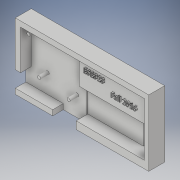
# Autodesk Inventor part: case2
Saved by Autodesk Inventor 2017 (Build 210142000, 142)
## iProperties
Created: 2016-12-01
Part Number: case2
Material: Generic
Document SubType Name: Modeling
Designer: SDL
Density: 1 g/cm^3
Appearance: Default
Author: SDL
Autodesk Inventor part; units mm, degrees
ref_plane "YZ Plane" through (0, 0, 0) normal (1, 0, 0) x (0, 1, 0)
ref_plane "XZ Plane" through (0, 0, 0) normal (0, 1, 0) x (-1, 0, 0)
ref_plane "XY Plane" through (0, 0, 0) normal (0, 0, 1) x (1, 0, 0)
sketch "Sketch3" plane through (0, 0, 0) normal (0, 0, 1) x (1, 0, 0)
  line L0 (0, 0) -> (125, 0)
  line L1 (125, 0) -> (125, 62)
  line L2 (125, 62) -> (0, 62)
  line L3 (0, 62) -> (0, 0)
  dimension "d0" = 125
  dimension "d1" = 62
  constraints: 8 end point, 2 parallel, 1 horizontal, 1 perpendicular
  measures "d0" distance of L2.end L1.end
  measures "d1" distance of L1.end L0.end
extrude "Extrusion1" add sketch "Sketch3" along normal blind 15
sketch "Sketch4" plane through (0, 0, 15) normal (0, 0, 1) x (1, 0, 0)
  line L0 (0, 62) -> (0, 0) projected
  line L1 (125, 0) -> (125, 62) projected
  line L2 (5, 57) -> (57, 57)
  line L3 (57, 57) -> (57, 5)
  line L4 (57, 5) -> (5, 5)
  line L5 (5, 5) -> (5, 57)
  line L6 (4, 57) -> (56, 5) construction
  line L7 (56, 57) -> (4, 5) construction
  dimension "d4" = 52
  dimension "d5" = 52
  constraints: 12 end point, 2 parallel, 1 horizontal, 1 perpendicular
  measures "d4" distance of L3.end L4.end
  measures "d5" distance of L2.end L3.end
extrude "Extrusion2" cut sketch "Sketch4" against normal blind 10
sketch "Sketch5" plane through (0, 0, 15) normal (0, 0, 1) x (1, 0, 0)
  line L0 (57, 57) -> (57, 5) projected
  line L1 (57, 5) -> (57, 7)
  line L2 (0, 0) -> (125, 0) projected
  line L3 (57, 7) -> (121, 7)
  line L4 (121, 7) -> (121, 33.5)
  line L5 (121, 33.5) -> (57, 33.5)
  line L6 (57, 33.5) -> (57, 7)
  dimension "d9" = 2
  dimension "d10" = 64
  dimension "d11" = 26.5
  constraints: 10 end point, 2 parallel, 2 perpendicular, 1 horizontal
  measures "d9" distance of L0.end L1.end
  measures "d10" distance of L5.end L4.end
  measures "d11" distance of L4.end L3.end
extrude "Extrusion3" cut sketch "Sketch5" against normal blind 10
sketch "Sketch6" plane through (0, 0, 15) normal (0, 0, 1) x (1, 0, 0)
  line L0 (121, 7) -> (57, 7) projected
  line L1 (57, 33.5) -> (121, 33.5) projected
  line L2 (121, 7) -> (109, 7)
  line L3 (109, 7) -> (109, 33.5)
  line L4 (109, 33.5) -> (121, 33.5)
  line L5 (121, 33.5) -> (121, 7)
  point P0 (0, 0)
  dimension "d14" = 12
  constraints: 8 end point, 2 parallel, 1 horizontal, 1 perpendicular, 1 point on line
  measures "d14" distance of L3.end L4.end
extrude "Extrusion4" cut sketch "Sketch6" against normal blind 15
sketch "Sketch7" plane through (0, 0, 15) normal (0, 0, 1) x (1, 0, 0)
  line L0 (109, 7) -> (57, 7) projected
  line L1 (109, 33.5) -> (109, 7) projected
  line L2 (57, 7) -> (109, 7)
  line L3 (109, 7) -> (109, 33.5)
  line L4 (109, 33.5) -> (57, 33.5)
  line L5 (57, 33.5) -> (57, 7)
  point P0 (0, 0)
  constraints: 8 end point, 2 parallel, 1 horizontal, 1 perpendicular
extrude "Extrusion5" cut sketch "Sketch7" against normal blind 11
sketch "Sketch8" plane through (0, 0, 5) normal (0, 0, 1) x (1, 0, 0)
  line L0 (5, 57) -> (57, 57) projected
  line L1 (57, 5) -> (5, 5) projected
  line L2 (5, 5) -> (5, 57) projected
  line L3 (57, 7) -> (57, 33.5) projected
  line L4 (6, 56) -> (56, 6) construction
  line L5 (56, 56) -> (6, 6) construction
  line L6 (6, 6) -> (20.3, 6) construction
  circle A0 centre (10.4, 53) radius 1.5
  circle A1 centre (20.3, 22.7) radius 1.5
  circle A2 centre (47.9, 18.5) radius 1.5
  point P0 (0, 0)
  point P1 (31, 31)
  dimension "d19" = 50
  dimension "d20" = 50
  dimension "d28" = 3
  dimension "d29" = 3
  dimension "d30" = 3
  constraints: 6 end point, 3 centre point, 2 midpoint, 1 horizontal
  measures "d19" distance of L4.end L5.end
  measures "d20" distance of L5.start L4.end
  measures "d28" diameter of A0
  measures "d29" diameter of A1
  measures "d30" diameter of A2
extrude "Extrusion6" add sketch "Sketch8" along normal blind 8
sketch "Sketch9" plane through (0, 0, 15) normal (0, 0, 1) x (1, 0, 0)
  line L0 (57, 5) -> (5, 5) projected
  line L1 (5, 5) -> (35, 5)
  line L2 (0, 0) -> (125, 0) projected
  line L3 (35, 5) -> (57, 5)
  line L4 (57, 5) -> (57, 0)
  line L5 (57, 0) -> (35, 0)
  line L6 (35, 0) -> (35, 5)
  constraints: 10 end point, 2 parallel, 2 point on line, 1 horizontal, 1 perpendicular
extrude "Extrusion7" cut sketch "Sketch9" against normal blind 10
sketch "Sketch10" plane through (0, 0, 15) normal (0, 0, 1) x (1, 0, 0)
  line L0 (5, 5) -> (5, 57) projected
  line L1 (5, 57) -> (5, 20)
  line L2 (5, 20) -> (0, 20)
  line L3 (0, 62) -> (0, 0) projected
  line L4 (5, 20) -> (0, 20)
  line L5 (0, 20) -> (0, 5)
  line L6 (0, 5) -> (5, 5)
  line L7 (5, 5) -> (5, 20)
  dimension "d36" = 37
  constraints: 12 end point, 3 point on line, 2 parallel, 2 perpendicular, 1 horizontal
  measures "d36" distance of L0.end L1.end
extrude "Extrusion8" cut sketch "Sketch10" against normal blind 10
sketch "Sketch13" plane through (0, 0, 15) normal (0, 0, 1) x (1, 0, 0)
  line L0 (57, 57) -> (57, 33.5) projected
  line L1 (57, 57) -> (121, 57)
  line L2 (121, 7) -> (121, 33.5) projected
  line L3 (57, 33.5) -> (109, 33.5) projected
  line L4 (121, 57) -> (57, 57)
  line L5 (57, 57) -> (57, 33.5)
  line L6 (57, 33.5) -> (121, 33.5)
  line L7 (121, 33.5) -> (121, 57)
  point P0 (0, 0)
  constraints: 10 end point, 2 parallel, 2 perpendicular, 1 horizontal
extrude "Extrusion9" cut sketch "Sketch13" against normal blind 3
sketch "Sketch14" plane through (0, 0, 12) normal (0, 0, 1) x (1, 0, 0)
  line L0 (61.9045, 52.1131) -> (81.5918, 52.1131) construction
  line L1 (81.5918, 52.1131) -> (81.5918, 47.138) construction
  line L2 (81.5918, 47.138) -> (61.9045, 47.138) construction
  line L3 (61.9045, 47.138) -> (61.9045, 52.1131) construction
  line L4 (87.5293, 45.1674) -> (113.4964, 45.1674) construction
  line L5 (113.4964, 45.1674) -> (113.4964, 38.1257) construction
  line L6 (113.4964, 38.1257) -> (87.5293, 38.1257) construction
  line L7 (87.5293, 38.1257) -> (87.5293, 45.1674) construction
  spline S0 degree 2 poles (64.7873, 48.0985) (64.7873, 48.0393) (64.7754, 47.9525) (64.7439, 47.8973) (64.7005, 47.8697) (64.6729, 47.8697) knots 0 0 0 1 2 3 4 4 4
  line L8 (64.6729, 47.8697) -> (62.6656, 47.8697)
  spline S1 degree 2 poles (62.6656, 47.8697) (62.5946, 47.8697) (62.4605, 47.9683) (62.4605, 48.0945) knots 0 0 0 1 2 2 2
  line L9 (62.4605, 48.0945) -> (62.4605, 51.8252)
  spline S2 degree 2 poles (62.4605, 51.8252) (62.4605, 51.9514) (62.5946, 52.05) (62.6656, 52.05) knots 0 0 0 1 2 2 2
  line L10 (62.6656, 52.05) -> (64.6492, 52.05)
  spline S3 degree 2 poles (64.6492, 52.05) (64.6769, 52.05) (64.7163, 52.0224) (64.7439, 51.9672) (64.7597, 51.8804) (64.7597, 51.8134) knots 0 0 0 1 2 3 4 4 4
  spline S4 degree 2 poles (64.7597, 51.8134) (64.7597, 51.7582) (64.7439, 51.6675) (64.7163, 51.6162) (64.6769, 51.5886) (64.6492, 51.5886) knots 0 0 0 1 2 3 4 4 4
  line L11 (64.6492, 51.5886) -> (63.0166, 51.5886)
  line L12 (63.0166, 51.5886) -> (63.0166, 50.2754)
  line L13 (63.0166, 50.2754) -> (64.4166, 50.2754)
  spline S5 degree 2 poles (64.4166, 50.2754) (64.4442, 50.2754) (64.4836, 50.2478) (64.5152, 50.1965) (64.527, 50.1058) (64.527, 50.0427) knots 0 0 0 1 2 3 4 4 4
  spline S6 degree 2 poles (64.527, 50.0427) (64.527, 49.9835) (64.5152, 49.9007) (64.4836, 49.8494) (64.4442, 49.8258) (64.4166, 49.8258) knots 0 0 0 1 2 3 4 4 4
  line L14 (64.4166, 49.8258) -> (63.0166, 49.8258)
  line L15 (63.0166, 49.8258) -> (63.0166, 48.3311)
  line L16 (63.0166, 48.3311) -> (64.6729, 48.3311)
  spline S7 degree 2 poles (64.6729, 48.3311) (64.7005, 48.3311) (64.7439, 48.3035) (64.7754, 48.2523) (64.7873, 48.1616) (64.7873, 48.0985) knots 0 0 0 1 2 3 4 4 4
  spline S8 degree 2 poles (67.9343, 49.041) (67.9343, 48.7492) (67.7174, 48.2878) (67.3349, 47.9683) (66.8143, 47.8066) (66.5146, 47.8066) knots 0 0 0 1 2 3 4 4 4
  spline S9 degree 2 poles (66.5146, 47.8066) (66.3016, 47.8066) (65.9428, 47.8776) (65.6628, 47.9801) (65.4735, 48.0906) (65.3985, 48.1655) (65.3631, 48.2838) (65.3631, 48.3863) knots 0 0 0 1 2 3 4 5 6 6 6
  spline S10 degree 2 poles (65.3631, 48.3863) (65.3631, 48.4573) (65.3749, 48.552) (65.4025, 48.6072) (65.4419, 48.6309) (65.4656, 48.6309) knots 0 0 0 1 2 3 4 4 4
  spline S11 degree 2 poles (65.4656, 48.6309) (65.5129, 48.6309) (65.6785, 48.5204) (65.9349, 48.3942) (66.3016, 48.2799) (66.5383, 48.2799) knots 0 0 0 1 2 3 4 4 4
  spline S12 degree 2 poles (66.5383, 48.2799) (66.7197, 48.2799) (67.0233, 48.3785) (67.2363, 48.5559) (67.3546, 48.8162) (67.3546, 48.9818) knots 0 0 0 1 2 3 4 4 4
  spline S13 degree 2 poles (67.3546, 48.9818) (67.3546, 49.1593) (67.1929, 49.4117) (66.9287, 49.601) (66.5895, 49.7587) (66.2307, 49.9244) (65.8954, 50.1255) (65.6312, 50.3976) (65.4656, 50.7604) (65.4656, 51.0168) knots 0 0 0 1 2 3 4 5 6 7 8 8 8
  spline S14 degree 2 poles (65.4656, 51.0168) (65.4656, 51.277) (65.6549, 51.6911) (65.994, 51.9672) (66.4633, 52.1131) (66.7354, 52.1131) knots 0 0 0 1 2 3 4 4 4
  spline S15 degree 2 poles (66.7354, 52.1131) (66.8735, 52.1131) (67.1535, 52.0658) (67.4019, 51.9869) (67.5991, 51.8844) (67.6583, 51.8252) (67.678, 51.7897) (67.6898, 51.7345) (67.6977, 51.6556) (67.6977, 51.5965) knots 0 0 0 1 2 3 4 5 6 7 8 8 8
  spline S16 degree 2 poles (67.6977, 51.5965) (67.6977, 51.5373) (67.6898, 51.4466) (67.6701, 51.3835) (67.6346, 51.3559) (67.6109, 51.3559) knots 0 0 0 1 2 3 4 4 4
  spline S17 degree 2 poles (67.6109, 51.3559) (67.5754, 51.3559) (67.4216, 51.4466) (67.2047, 51.557) (66.9011, 51.6517) (66.7157, 51.6517) knots 0 0 0 1 2 3 4 4 4
  spline S18 degree 2 poles (66.7157, 51.6517) (66.5422, 51.6517) (66.2819, 51.557) (66.1123, 51.4032) (66.0295, 51.1903) (66.0295, 51.068) knots 0 0 0 1 2 3 4 4 4
  spline S19 degree 2 poles (66.0295, 51.068) (66.0295, 50.8945) (66.1912, 50.6421) (66.4594, 50.4489) (66.8025, 50.2872) (67.1574, 50.1216) (67.5005, 49.9244) (67.7687, 49.6562) (67.9343, 49.2894) (67.9343, 49.041) knots 0 0 0 1 2 3 4 5 6 7 8 8 8
  spline S20 degree 2 poles (71.0577, 48.0985) (71.0577, 48.0393) (71.0459, 47.9525) (71.0143, 47.8973) (70.9709, 47.8697) (70.9433, 47.8697) knots 0 0 0 1 2 3 4 4 4
  line L17 (70.9433, 47.8697) -> (68.936, 47.8697)
  spline S21 degree 2 poles (68.936, 47.8697) (68.865, 47.8697) (68.7309, 47.9683) (68.7309, 48.0945) knots 0 0 0 1 2 2 2
  line L18 (68.7309, 48.0945) -> (68.7309, 51.8252)
  spline S22 degree 2 poles (68.7309, 51.8252) (68.7309, 51.9514) (68.865, 52.05) (68.936, 52.05) knots 0 0 0 1 2 2 2
  line L19 (68.936, 52.05) -> (70.9197, 52.05)
  spline S23 degree 2 poles (70.9197, 52.05) (70.9473, 52.05) (70.9867, 52.0224) (71.0143, 51.9672) (71.0301, 51.8804) (71.0301, 51.8134) knots 0 0 0 1 2 3 4 4 4
  spline S24 degree 2 poles (71.0301, 51.8134) (71.0301, 51.7582) (71.0143, 51.6675) (70.9867, 51.6162) (70.9473, 51.5886) (70.9197, 51.5886) knots 0 0 0 1 2 3 4 4 4
  line L20 (70.9197, 51.5886) -> (69.287, 51.5886)
  line L21 (69.287, 51.5886) -> (69.287, 50.2754)
  line L22 (69.287, 50.2754) -> (70.687, 50.2754)
  spline S25 degree 2 poles (70.687, 50.2754) (70.7146, 50.2754) (70.754, 50.2478) (70.7856, 50.1965) (70.7974, 50.1058) (70.7974, 50.0427) knots 0 0 0 1 2 3 4 4 4
  spline S26 degree 2 poles (70.7974, 50.0427) (70.7974, 49.9835) (70.7856, 49.9007) (70.754, 49.8494) (70.7146, 49.8258) (70.687, 49.8258) knots 0 0 0 1 2 3 4 4 4
  line L23 (70.687, 49.8258) -> (69.287, 49.8258)
  line L24 (69.287, 49.8258) -> (69.287, 48.3311)
  line L25 (69.287, 48.3311) -> (70.9433, 48.3311)
  spline S27 degree 2 poles (70.9433, 48.3311) (70.9709, 48.3311) (71.0143, 48.3035) (71.0459, 48.2523) (71.0577, 48.1616) (71.0577, 48.0985) knots 0 0 0 1 2 3 4 4 4
  spline S28 degree 2 poles (74.3546, 49.0647) (74.3546, 48.7768) (74.1535, 48.3154) (73.7788, 47.9841) (73.2307, 47.8066) (72.8836, 47.8066) knots 0 0 0 1 2 3 4 4 4
  spline S29 degree 2 poles (72.8836, 47.8066) (72.6746, 47.8066) (72.3118, 47.8737) (72.0278, 47.9683) (71.8385, 48.0669) (71.7912, 48.1142) (71.7636, 48.1576) (71.7439, 48.2247) (71.736, 48.3154) (71.736, 48.3863) knots 0 0 0 1 2 3 4 5 6 7 8 8 8
  spline S30 degree 2 poles (71.736, 48.3863) (71.736, 48.5007) (71.7833, 48.5914) (71.8267, 48.5914) knots 0 0 0 1 2 2 2
  spline S31 degree 2 poles (71.8267, 48.5914) (71.8543, 48.5914) (72.0318, 48.4889) (72.3039, 48.3666) (72.6746, 48.2641) (72.8994, 48.2641) knots 0 0 0 1 2 3 4 4 4
  spline S32 degree 2 poles (72.8994, 48.2641) (73.1163, 48.2641) (73.4476, 48.3745) (73.6723, 48.5756) (73.7867, 48.8478) (73.7867, 49.0094) knots 0 0 0 1 2 3 4 4 4
  spline S33 degree 2 poles (73.7867, 49.0094) (73.7867, 49.1909) (73.6447, 49.4748) (73.3647, 49.6799) (72.9625, 49.7903) (72.7061, 49.7903) knots 0 0 0 1 2 3 4 4 4
  line L26 (72.7061, 49.7903) -> (72.296, 49.7903)
  spline S34 degree 2 poles (72.296, 49.7903) (72.2684, 49.7903) (72.2171, 49.814) (72.1816, 49.8652) (72.158, 49.948) (72.158, 50.0151) knots 0 0 0 1 2 3 4 4 4
  spline S35 degree 2 poles (72.158, 50.0151) (72.158, 50.0782) (72.1777, 50.157) (72.2132, 50.2044) (72.2566, 50.228) (72.2881, 50.228) knots 0 0 0 1 2 3 4 4 4
  line L27 (72.2881, 50.228) -> (72.6509, 50.228)
  spline S36 degree 2 poles (72.6509, 50.228) (72.8639, 50.228) (73.2031, 50.3385) (73.4397, 50.5475) (73.5659, 50.8354) (73.5659, 51.0128) knots 0 0 0 1 2 3 4 4 4
  spline S37 degree 2 poles (73.5659, 51.0128) (73.5659, 51.143) (73.4831, 51.3796) (73.3135, 51.557) (73.0532, 51.6556) (72.8797, 51.6556) knots 0 0 0 1 2 3 4 4 4
  spline S38 degree 2 poles (72.8797, 51.6556) (72.6943, 51.6556) (72.3788, 51.5413) (72.1343, 51.4151) (71.9726, 51.3007) (71.9411, 51.3007) knots 0 0 0 1 2 3 4 4 4
  spline S39 degree 2 poles (71.9411, 51.3007) (71.9174, 51.3007) (71.8819, 51.3165) (71.8583, 51.3638) (71.8504, 51.4506) (71.8504, 51.5216) knots 0 0 0 1 2 3 4 4 4
  spline S40 degree 2 poles (71.8504, 51.5216) (71.8504, 51.5728) (71.8583, 51.6438) (71.878, 51.699) (71.9016, 51.7463) (71.9647, 51.8055) (72.1501, 51.9238) (72.4261, 52.0342) (72.785, 52.1131) (72.9901, 52.1131) knots 0 0 0 1 2 3 4 5 6 7 8 8 8
  spline S41 degree 2 poles (72.9901, 52.1131) (73.2819, 52.1131) (73.7236, 51.9632) (74.0154, 51.6911) (74.1614, 51.3125) (74.1614, 51.0838) knots 0 0 0 1 2 3 4 4 4
  spline S42 degree 2 poles (74.1614, 51.0838) (74.1614, 50.8866) (74.0588, 50.5475) (73.8577, 50.2832) (73.5659, 50.0979) (73.3766, 50.0624) knots 0 0 0 1 2 3 4 4 4
  line L28 (73.3766, 50.0624) -> (73.3766, 50.0585)
  spline S43 degree 2 poles (73.3766, 50.0585) (73.5935, 50.0348) (73.9523, 49.8652) (74.2087, 49.6049) (74.3546, 49.2579) (74.3546, 49.0647) knots 0 0 0 1 2 3 4 4 4
  spline S44 degree 2 poles (77.7422, 48.1103) (77.7422, 48.0511) (77.7264, 47.9604) (77.6988, 47.8973) (77.6476, 47.8697) (77.62, 47.8697) knots 0 0 0 1 2 3 4 4 4
  line L29 (77.62, 47.8697) -> (75.309, 47.8697)
  spline S45 degree 2 poles (75.309, 47.8697) (75.2616, 47.8697) (75.1946, 47.8934) (75.1473, 47.9447) (75.1236, 48.0432) (75.1236, 48.1142) knots 0 0 0 1 2 3 4 4 4
  spline S46 degree 2 poles (75.1236, 48.1142) (75.1236, 48.1773) (75.1354, 48.2759) (75.167, 48.3509) (75.2183, 48.4218) (75.2577, 48.4652) knots 0 0 0 1 2 3 4 4 4
  line L30 (75.2577, 48.4652) -> (76.0938, 49.3249)
  spline S47 degree 2 poles (76.0938, 49.3249) (76.3856, 49.6207) (76.7366, 50.094) (76.9259, 50.4804) (76.985, 50.7959) (76.985, 50.9379) knots 0 0 0 1 2 3 4 4 4
  spline S48 degree 2 poles (76.985, 50.9379) (76.985, 51.0759) (76.8904, 51.3244) (76.7129, 51.5097) (76.4487, 51.6201) (76.2752, 51.6201) knots 0 0 0 1 2 3 4 4 4
  spline S49 degree 2 poles (76.2752, 51.6201) (76.0701, 51.6201) (75.7467, 51.5097) (75.5022, 51.3835) (75.3405, 51.2731) (75.3011, 51.2731) knots 0 0 0 1 2 3 4 4 4
  spline S50 degree 2 poles (75.3011, 51.2731) (75.2774, 51.2731) (75.238, 51.3007) (75.2143, 51.3559) (75.2025, 51.4545) (75.2025, 51.5216) knots 0 0 0 1 2 3 4 4 4
  spline S51 degree 2 poles (75.2025, 51.5216) (75.2025, 51.5689) (75.2104, 51.6399) (75.2261, 51.6951) (75.2498, 51.7385) (75.3287, 51.8055) (75.518, 51.9238) (75.8059, 52.0342) (76.1529, 52.1131) (76.3422, 52.1131) knots 0 0 0 1 2 3 4 5 6 7 8 8 8
  spline S52 degree 2 poles (76.3422, 52.1131) (76.6459, 52.1131) (77.1033, 51.9435) (77.4031, 51.6438) (77.5529, 51.2494) (77.5529, 51.0286) knots 0 0 0 1 2 3 4 4 4
  spline S53 degree 2 poles (77.5529, 51.0286) (77.5529, 50.8275) (77.4819, 50.4292) (77.2532, 49.9678) (76.8194, 49.4038) (76.4566, 49.0331) knots 0 0 0 1 2 3 4 4 4
  line L31 (76.4566, 49.0331) -> (75.794, 48.343)
  line L32 (75.794, 48.343) -> (77.616, 48.343)
  spline S54 degree 2 poles (77.616, 48.343) (77.6436, 48.343) (77.6909, 48.3154) (77.7264, 48.2562) (77.7422, 48.1694) (77.7422, 48.1103) knots 0 0 0 1 2 3 4 4 4
  spline S55 degree 2 poles (81.0588, 49.0647) (81.0588, 48.7768) (80.8577, 48.3154) (80.4831, 47.9841) (79.9349, 47.8066) (79.5878, 47.8066) knots 0 0 0 1 2 3 4 4 4
  spline S56 degree 2 poles (79.5878, 47.8066) (79.3788, 47.8066) (79.016, 47.8737) (78.7321, 47.9683) (78.5428, 48.0669) (78.4954, 48.1142) (78.4678, 48.1576) (78.4481, 48.2247) (78.4402, 48.3154) (78.4402, 48.3863) knots 0 0 0 1 2 3 4 5 6 7 8 8 8
  spline S57 degree 2 poles (78.4402, 48.3863) (78.4402, 48.5007) (78.4876, 48.5914) (78.5309, 48.5914) knots 0 0 0 1 2 2 2
  spline S58 degree 2 poles (78.5309, 48.5914) (78.5585, 48.5914) (78.736, 48.4889) (79.0081, 48.3666) (79.3788, 48.2641) (79.6036, 48.2641) knots 0 0 0 1 2 3 4 4 4
  spline S59 degree 2 poles (79.6036, 48.2641) (79.8205, 48.2641) (80.1518, 48.3745) (80.3766, 48.5756) (80.4909, 48.8478) (80.4909, 49.0094) knots 0 0 0 1 2 3 4 4 4
  spline S60 degree 2 poles (80.4909, 49.0094) (80.4909, 49.1909) (80.349, 49.4748) (80.069, 49.6799) (79.6667, 49.7903) (79.4104, 49.7903) knots 0 0 0 1 2 3 4 4 4
  line L33 (79.4104, 49.7903) -> (79.0002, 49.7903)
  spline S61 degree 2 poles (79.0002, 49.7903) (78.9726, 49.7903) (78.9214, 49.814) (78.8859, 49.8652) (78.8622, 49.948) (78.8622, 50.0151) knots 0 0 0 1 2 3 4 4 4
  spline S62 degree 2 poles (78.8622, 50.0151) (78.8622, 50.0782) (78.8819, 50.157) (78.9174, 50.2044) (78.9608, 50.228) (78.9923, 50.228) knots 0 0 0 1 2 3 4 4 4
  line L34 (78.9923, 50.228) -> (79.3552, 50.228)
  spline S63 degree 2 poles (79.3552, 50.228) (79.5681, 50.228) (79.9073, 50.3385) (80.1439, 50.5475) (80.2701, 50.8354) (80.2701, 51.0128) knots 0 0 0 1 2 3 4 4 4
  spline S64 degree 2 poles (80.2701, 51.0128) (80.2701, 51.143) (80.1873, 51.3796) (80.0177, 51.557) (79.7574, 51.6556) (79.5839, 51.6556) knots 0 0 0 1 2 3 4 4 4
  spline S65 degree 2 poles (79.5839, 51.6556) (79.3985, 51.6556) (79.0831, 51.5413) (78.8385, 51.4151) (78.6769, 51.3007) (78.6453, 51.3007) knots 0 0 0 1 2 3 4 4 4
  spline S66 degree 2 poles (78.6453, 51.3007) (78.6216, 51.3007) (78.5861, 51.3165) (78.5625, 51.3638) (78.5546, 51.4506) (78.5546, 51.5216) knots 0 0 0 1 2 3 4 4 4
  spline S67 degree 2 poles (78.5546, 51.5216) (78.5546, 51.5728) (78.5625, 51.6438) (78.5822, 51.699) (78.6059, 51.7463) (78.669, 51.8055) (78.8543, 51.9238) (79.1304, 52.0342) (79.4892, 52.1131) (79.6943, 52.1131) knots 0 0 0 1 2 3 4 5 6 7 8 8 8
  spline S68 degree 2 poles (79.6943, 52.1131) (79.9861, 52.1131) (80.4278, 51.9632) (80.7197, 51.6911) (80.8656, 51.3125) (80.8656, 51.0838) knots 0 0 0 1 2 3 4 4 4
  spline S69 degree 2 poles (80.8656, 51.0838) (80.8656, 50.8866) (80.7631, 50.5475) (80.5619, 50.2832) (80.2701, 50.0979) (80.0808, 50.0624) knots 0 0 0 1 2 3 4 4 4
  line L35 (80.0808, 50.0624) -> (80.0808, 50.0585)
  spline S70 degree 2 poles (80.0808, 50.0585) (80.2977, 50.0348) (80.6566, 49.8652) (80.9129, 49.6049) (81.0588, 49.2579) (81.0588, 49.0647) knots 0 0 0 1 2 3 4 4 4
  spline S71 degree 2 poles (90.282, 44.6074) (90.282, 44.5483) (90.2701, 44.4576) (90.2386, 44.4024) (90.1952, 44.3748) (90.1716, 44.3748) knots 0 0 0 1 2 3 4 4 4
  line L36 (90.1716, 44.3748) -> (88.6414, 44.3748)
  line L37 (88.6414, 44.3748) -> (88.6414, 42.955)
  line L38 (88.6414, 42.955) -> (90.0887, 42.955)
  spline S72 degree 2 poles (90.0887, 42.955) (90.1124, 42.955) (90.1518, 42.9314) (90.1834, 42.8801) (90.1992, 42.7934) (90.1992, 42.7263) knots 0 0 0 1 2 3 4 4 4
  spline S73 degree 2 poles (90.1992, 42.7263) (90.1992, 42.6632) (90.1834, 42.5765) (90.1518, 42.5212) (90.1124, 42.4936) (90.0887, 42.4936) knots 0 0 0 1 2 3 4 4 4
  line L39 (90.0887, 42.4936) -> (88.6414, 42.4936)
  line L40 (88.6414, 42.4936) -> (88.6414, 40.7505)
  spline S74 degree 2 poles (88.6414, 40.7505) (88.6414, 40.7269) (88.6138, 40.6874) (88.5507, 40.6638) (88.4482, 40.648) (88.3654, 40.648) knots 0 0 0 1 2 3 4 4 4
  spline S75 degree 2 poles (88.3654, 40.648) (88.2865, 40.648) (88.1761, 40.6638) (88.113, 40.6874) (88.0854, 40.7269) (88.0854, 40.7505) knots 0 0 0 1 2 3 4 4 4
  line L41 (88.0854, 40.7505) -> (88.0854, 44.6232)
  spline S76 degree 2 poles (88.0854, 44.6232) (88.0854, 44.7494) (88.2194, 44.848) (88.2904, 44.848) knots 0 0 0 1 2 2 2
  line L42 (88.2904, 44.848) -> (90.1716, 44.848)
  spline S77 degree 2 poles (90.1716, 44.848) (90.1952, 44.848) (90.2386, 44.8204) (90.2701, 44.7652) (90.282, 44.6705) (90.282, 44.6074) knots 0 0 0 1 2 3 4 4 4
  spline S78 degree 2 poles (93.2516, 40.7466) (93.2516, 40.7072) (93.2003, 40.6677) (93.1096, 40.648) (93.0228, 40.648) knots 0 0 0 1 2 3 3 3
  spline S79 degree 2 poles (93.0228, 40.648) (92.94, 40.648) (92.8375, 40.6677) (92.7941, 40.7072) (92.7941, 40.7466) knots 0 0 0 1 2 3 3 3
  line L43 (92.7941, 40.7466) -> (92.7941, 41.0345)
  spline S80 degree 2 poles (92.7941, 41.0345) (92.6048, 40.8334) (92.1355, 40.6046) (91.8752, 40.6046) knots 0 0 0 1 2 2 2
  spline S81 degree 2 poles (91.8752, 40.6046) (91.6425, 40.6046) (91.2718, 40.7229) (91.0116, 40.9517) (90.8656, 41.2829) (90.8656, 41.4919) knots 0 0 0 1 2 3 4 4 4
  spline S82 degree 2 poles (90.8656, 41.4919) (90.8656, 41.7404) (91.0668, 42.1032) (91.4414, 42.3438) (91.9817, 42.4621) (92.3208, 42.4621) knots 0 0 0 1 2 3 4 4 4
  line L44 (92.3208, 42.4621) -> (92.7231, 42.4621)
  line L45 (92.7231, 42.4621) -> (92.7231, 42.6869)
  spline S83 degree 2 poles (92.7231, 42.6869) (92.7231, 42.8565) (92.6521, 43.1128) (92.4944, 43.2824) (92.242, 43.3691) (92.0566, 43.3691) knots 0 0 0 1 2 3 4 4 4
  spline S84 degree 2 poles (92.0566, 43.3691) (91.8594, 43.3691) (91.5479, 43.2745) (91.3113, 43.1641) (91.1535, 43.0694) (91.1141, 43.0694) knots 0 0 0 1 2 3 4 4 4
  spline S85 degree 2 poles (91.1141, 43.0694) (91.0865, 43.0694) (91.051, 43.097) (91.0194, 43.1483) (91.0076, 43.2272) (91.0076, 43.2745) knots 0 0 0 1 2 3 4 4 4
  spline S86 degree 2 poles (91.0076, 43.2745) (91.0076, 43.3573) (91.0313, 43.4519) (91.118, 43.5348) (91.331, 43.6491) (91.607, 43.7398) (91.9383, 43.8029) (92.1039, 43.8029) knots 0 0 0 1 2 3 4 5 6 6 6
  spline S87 degree 2 poles (92.1039, 43.8029) (92.4194, 43.8029) (92.8572, 43.661) (93.1293, 43.3849) (93.2516, 42.9787) (93.2516, 42.7066) knots 0 0 0 1 2 3 4 4 4
  line L46 (93.2516, 42.7066) -> (93.2516, 40.7466)
  line L47 (92.7231, 42.0756) -> (92.2656, 42.0756)
  spline S88 degree 2 poles (92.2656, 42.0756) (92.0487, 42.0756) (91.7254, 42.0007) (91.5085, 41.8548) (91.4099, 41.6497) (91.4099, 41.5196) knots 0 0 0 1 2 3 4 4 4
  spline S89 degree 2 poles (91.4099, 41.5196) (91.4099, 41.2908) (91.6977, 41.0227) (91.958, 41.0227) knots 0 0 0 1 2 2 2
  spline S90 degree 2 poles (91.958, 41.0227) (92.167, 41.0227) (92.5259, 41.2356) (92.7231, 41.4565) knots 0 0 0 1 2 2 2
  line L48 (92.7231, 41.4565) -> (92.7231, 42.0756)
  spline S91 degree 2 poles (94.7659, 40.7466) (94.7659, 40.7229) (94.7383, 40.6874) (94.6831, 40.6598) (94.5806, 40.648) (94.4977, 40.648) knots 0 0 0 1 2 3 4 4 4
  spline S92 degree 2 poles (94.4977, 40.648) (94.4189, 40.648) (94.3163, 40.6598) (94.2572, 40.6874) (94.2335, 40.7229) (94.2335, 40.7466) knots 0 0 0 1 2 3 4 4 4
  line L49 (94.2335, 40.7466) -> (94.2335, 45.0649)
  spline S93 degree 2 poles (94.2335, 45.0649) (94.2335, 45.0886) (94.2572, 45.128) (94.3163, 45.1556) (94.4189, 45.1674) (94.4977, 45.1674) knots 0 0 0 1 2 3 4 4 4
  spline S94 degree 2 poles (94.4977, 45.1674) (94.5806, 45.1674) (94.6831, 45.1556) (94.7383, 45.128) (94.7659, 45.0886) (94.7659, 45.0649) knots 0 0 0 1 2 3 4 4 4
  line L50 (94.7659, 45.0649) -> (94.7659, 40.7466)
  spline S95 degree 2 poles (96.2842, 40.7466) (96.2842, 40.7229) (96.2566, 40.6874) (96.2014, 40.6598) (96.0989, 40.648) (96.0161, 40.648) knots 0 0 0 1 2 3 4 4 4
  spline S96 degree 2 poles (96.0161, 40.648) (95.9372, 40.648) (95.8346, 40.6598) (95.7755, 40.6874) (95.7518, 40.7229) (95.7518, 40.7466) knots 0 0 0 1 2 3 4 4 4
  line L51 (95.7518, 40.7466) -> (95.7518, 45.0649)
  spline S97 degree 2 poles (95.7518, 45.0649) (95.7518, 45.0886) (95.7755, 45.128) (95.8346, 45.1556) (95.9372, 45.1674) (96.0161, 45.1674) knots 0 0 0 1 2 3 4 4 4
  spline S98 degree 2 poles (96.0161, 45.1674) (96.0989, 45.1674) (96.2014, 45.1556) (96.2566, 45.128) (96.2842, 45.0886) (96.2842, 45.0649) knots 0 0 0 1 2 3 4 4 4
  line L52 (96.2842, 45.0649) -> (96.2842, 40.7466)
  spline S99 degree 2 poles (101.2572, 40.9083) (101.2572, 40.8491) (101.2414, 40.7584) (101.2138, 40.6953) (101.1625, 40.6677) (101.1349, 40.6677) knots 0 0 0 1 2 3 4 4 4
  line L53 (101.1349, 40.6677) -> (98.8239, 40.6677)
  spline S100 degree 2 poles (98.8239, 40.6677) (98.7766, 40.6677) (98.7096, 40.6914) (98.6623, 40.7427) (98.6386, 40.8412) (98.6386, 40.9122) knots 0 0 0 1 2 3 4 4 4
  spline S101 degree 2 poles (98.6386, 40.9122) (98.6386, 40.9753) (98.6504, 41.0739) (98.682, 41.1488) (98.7332, 41.2198) (98.7727, 41.2632) knots 0 0 0 1 2 3 4 4 4
  line L54 (98.7727, 41.2632) -> (99.6087, 42.1229)
  spline S102 degree 2 poles (99.6087, 42.1229) (99.9006, 42.4187) (100.2516, 42.8919) (100.4408, 43.2784) (100.5, 43.5939) (100.5, 43.7359) knots 0 0 0 1 2 3 4 4 4
  spline S103 degree 2 poles (100.5, 43.7359) (100.5, 43.8739) (100.4054, 44.1224) (100.2279, 44.3077) (99.9637, 44.4181) (99.7901, 44.4181) knots 0 0 0 1 2 3 4 4 4
  spline S104 degree 2 poles (99.7901, 44.4181) (99.5851, 44.4181) (99.2617, 44.3077) (99.0172, 44.1815) (98.8555, 44.0711) (98.8161, 44.0711) knots 0 0 0 1 2 3 4 4 4
  spline S105 degree 2 poles (98.8161, 44.0711) (98.7924, 44.0711) (98.753, 44.0987) (98.7293, 44.1539) (98.7175, 44.2525) (98.7175, 44.3196) knots 0 0 0 1 2 3 4 4 4
  spline S106 degree 2 poles (98.7175, 44.3196) (98.7175, 44.3669) (98.7254, 44.4379) (98.7411, 44.4931) (98.7648, 44.5365) (98.8437, 44.6035) (99.033, 44.7218) (99.3208, 44.8322) (99.6679, 44.9111) (99.8572, 44.9111) knots 0 0 0 1 2 3 4 5 6 7 8 8 8
  spline S107 degree 2 poles (99.8572, 44.9111) (100.1608, 44.9111) (100.6183, 44.7415) (100.918, 44.4418) (101.0679, 44.0474) (101.0679, 43.8266) knots 0 0 0 1 2 3 4 4 4
  spline S108 degree 2 poles (101.0679, 43.8266) (101.0679, 43.6255) (100.9969, 43.2272) (100.7682, 42.7657) (100.3344, 42.2018) (99.9716, 41.8311) knots 0 0 0 1 2 3 4 4 4
  line L55 (99.9716, 41.8311) -> (99.309, 41.141)
  line L56 (99.309, 41.141) -> (101.131, 41.141)
  spline S109 degree 2 poles (101.131, 41.141) (101.1586, 41.141) (101.2059, 41.1134) (101.2414, 41.0542) (101.2572, 40.9674) (101.2572, 40.9083) knots 0 0 0 1 2 3 4 4 4
  spline S110 degree 2 poles (104.7473, 42.7657) (104.7473, 42.2846) (104.5975, 41.4919) (104.2425, 40.9201) (103.6746, 40.6046) (103.2566, 40.6046) knots 0 0 0 1 2 3 4 4 4
  spline S111 degree 2 poles (103.2566, 40.6046) (102.8662, 40.6046) (102.3259, 40.8846) (101.9946, 41.4328) (101.8566, 42.2294) (101.8566, 42.75) knots 0 0 0 1 2 3 4 4 4
  spline S112 degree 2 poles (101.8566, 42.75) (101.8566, 43.2272) (102.0104, 44.0238) (102.3614, 44.5956) (102.9293, 44.9111) (103.3434, 44.9111) knots 0 0 0 1 2 3 4 4 4
  spline S113 degree 2 poles (103.3434, 44.9111) (103.7377, 44.9111) (104.278, 44.6311) (104.6093, 44.0829) (104.7473, 43.2863) (104.7473, 42.7657) knots 0 0 0 1 2 3 4 4 4
  spline S114 degree 2 poles (104.1794, 42.7303) (104.1794, 43.0418) (104.1361, 43.5387) (104.0454, 43.9212) (103.9073, 44.1934) (103.7141, 44.3748) (103.4656, 44.4536) (103.3118, 44.4536) knots 0 0 0 1 2 3 4 5 6 6 6
  spline S115 degree 2 poles (103.3118, 44.4536) (103.0358, 44.4536) (102.6927, 44.1934) (102.4955, 43.7438) (102.4245, 43.1365) (102.4245, 42.7855) knots 0 0 0 1 2 3 4 4 4
  spline S116 degree 2 poles (102.4245, 42.7855) (102.4245, 42.3201) (102.5231, 41.6615) (102.7321, 41.2514) (103.0594, 41.0621) (103.2921, 41.0621) knots 0 0 0 1 2 3 4 4 4
  spline S117 degree 2 poles (103.2921, 41.0621) (103.4735, 41.0621) (103.7456, 41.1765) (103.9428, 41.3934) (104.073, 41.697) (104.1518, 42.0677) (104.1794, 42.4976) (104.1794, 42.7303) knots 0 0 0 1 2 3 4 5 6 6 6
  spline S118 degree 2 poles (107.9693, 40.8886) (107.9693, 40.8255) (107.9496, 40.7427) (107.918, 40.6914) (107.8746, 40.6677) (107.8549, 40.6677) knots 0 0 0 1 2 3 4 4 4
  line L57 (107.8549, 40.6677) -> (105.6701, 40.6677)
  spline S119 degree 2 poles (105.6701, 40.6677) (105.6465, 40.6677) (105.607, 40.6914) (105.5716, 40.7427) (105.5518, 40.8255) (105.5518, 40.8886) knots 0 0 0 1 2 3 4 4 4
  spline S120 degree 2 poles (105.5518, 40.8886) (105.5518, 40.9438) (105.5716, 41.0305) (105.5992, 41.0857) (105.6425, 41.1134) (105.6701, 41.1134) knots 0 0 0 1 2 3 4 4 4
  line L58 (105.6701, 41.1134) -> (106.5417, 41.1134)
  line L59 (106.5417, 41.1134) -> (106.5417, 44.2959)
  line L60 (106.5417, 44.2959) -> (105.7332, 43.8148)
  spline S121 degree 2 poles (105.7332, 43.8148) (105.6701, 43.7832) (105.5992, 43.7714) (105.5518, 43.8108) (105.5361, 43.9094) (105.5361, 43.9843) knots 0 0 0 1 2 3 4 4 4
  spline S122 degree 2 poles (105.5361, 43.9843) (105.5361, 44.0356) (105.5439, 44.1145) (105.5637, 44.1657) (105.5992, 44.2052) (105.6307, 44.2249) knots 0 0 0 1 2 3 4 4 4
  line L61 (105.6307, 44.2249) -> (106.593, 44.8401)
  spline S123 degree 2 poles (106.593, 44.8401) (106.6048, 44.8519) (106.6442, 44.8638) (106.7034, 44.8756) (106.7823, 44.8796) (106.8375, 44.8796) knots 0 0 0 1 2 3 4 4 4
  spline S124 degree 2 poles (106.8375, 44.8796) (106.9163, 44.8796) (107.0189, 44.8677) (107.078, 44.8441) (107.0977, 44.8086) (107.0977, 44.7888) knots 0 0 0 1 2 3 4 4 4
  line L62 (107.0977, 44.7888) -> (107.0977, 41.1134)
  line L63 (107.0977, 41.1134) -> (107.8549, 41.1134)
  spline S125 degree 2 poles (107.8549, 41.1134) (107.8786, 41.1134) (107.9259, 41.0857) (107.9535, 41.0305) (107.9693, 40.9438) (107.9693, 40.8886) knots 0 0 0 1 2 3 4 4 4
  spline S126 degree 2 poles (111.42, 42.0204) (111.42, 41.7443) (111.2504, 41.2317) (110.9034, 40.8412) (110.367, 40.6046) (110.0042, 40.6046) knots 0 0 0 1 2 3 4 4 4
  spline S127 degree 2 poles (110.0042, 40.6046) (109.74, 40.6046) (109.3417, 40.7348) (109.042, 40.9714) (108.8448, 41.3224) (108.7265, 41.768) (108.6752, 42.3004) (108.6752, 42.6041) knots 0 0 0 1 2 3 4 5 6 6 6
  spline S128 degree 2 poles (108.6752, 42.6041) (108.6752, 42.8722) (108.7344, 43.4204) (108.8803, 43.9291) (109.1366, 44.3787) (109.5231, 44.7139) (110.0594, 44.9072) (110.4144, 44.9072) knots 0 0 0 1 2 3 4 5 6 6 6
  spline S129 degree 2 poles (110.4144, 44.9072) (110.5327, 44.9072) (110.7772, 44.8796) (110.9862, 44.8283) (111.1282, 44.7731) (111.1716, 44.7376) (111.1952, 44.6942) (111.207, 44.6469) (111.2149, 44.5838) (111.2149, 44.5404) knots 0 0 0 1 2 3 4 5 6 7 8 8 8
  spline S130 degree 2 poles (111.2149, 44.5404) (111.2149, 44.4812) (111.211, 44.3984) (111.1873, 44.3472) (111.1518, 44.3196) (111.1242, 44.3196) knots 0 0 0 1 2 3 4 4 4
  spline S131 degree 2 poles (111.1242, 44.3196) (111.0887, 44.3196) (110.9665, 44.3669) (110.793, 44.4221) (110.5445, 44.4655) (110.3789, 44.4655) knots 0 0 0 1 2 3 4 4 4
  spline S132 degree 2 poles (110.3789, 44.4655) (110.0792, 44.4655) (109.6454, 44.221) (109.3732, 43.8029) (109.2392, 43.2587) (109.2313, 42.959) knots 0 0 0 1 2 3 4 4 4
  spline S133 degree 2 poles (109.2313, 42.959) (109.3141, 43.0063) (109.5231, 43.1049) (109.7716, 43.1838) (110.0476, 43.2311) (110.2054, 43.2311) knots 0 0 0 1 2 3 4 4 4
  spline S134 degree 2 poles (110.2054, 43.2311) (110.5445, 43.2311) (111.0099, 43.0457) (111.2977, 42.7224) (111.42, 42.2767) (111.42, 42.0204) knots 0 0 0 1 2 3 4 4 4
  spline S135 degree 2 poles (110.8561, 41.9691) (110.8561, 42.1584) (110.7811, 42.4621) (110.6076, 42.675) (110.3197, 42.7934) (110.1068, 42.7934) knots 0 0 0 1 2 3 4 4 4
  spline S136 degree 2 poles (110.1068, 42.7934) (109.9845, 42.7934) (109.7479, 42.75) (109.527, 42.675) (109.322, 42.5765) (109.2392, 42.5173) knots 0 0 0 1 2 3 4 4 4
  spline S137 degree 2 poles (109.2392, 42.5173) (109.2392, 42.1032) (109.3456, 41.5393) (109.5468, 41.2001) (109.8504, 41.0542) (110.0555, 41.0542) knots 0 0 0 1 2 3 4 4 4
  spline S138 degree 2 poles (110.0555, 41.0542) (110.2606, 41.0542) (110.5642, 41.208) (110.7614, 41.4722) (110.8561, 41.7996) (110.8561, 41.9691) knots 0 0 0 1 2 3 4 4 4
  point P0 (0, 0)
  constraints: 4 other
extrude "Extrusion10" add sketch "Sketch14" along normal blind 1.5
body "Solid1"
